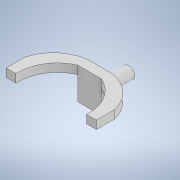
# Autodesk Inventor part: End
Saved by Autodesk Inventor 2022 (Build 260153000, 153)
## iProperties
Created: 2022-01-28
Part Number: End
Material: Generic
Document SubType Name: Modeling
Designer: Alexa
Density: 1 g/cm^3
Appearance: Default
Author: Alexa
Autodesk Inventor part; units mm, degrees
ref_plane "YZ Plane" through (0, 0, 0) normal (1, 0, 0) x (0, 1, 0)
ref_plane "XZ Plane" through (0, 0, 0) normal (0, 1, 0) x (-1, 0, 0)
ref_plane "XY Plane" through (0, 0, 0) normal (0, 0, 1) x (1, 0, 0)
sketch "Sketch1" plane through (0, 0, 0) normal (0, 0, 1) x (1, 0, 0)
  circle A0 centre (0, 0) radius 6
  dimension "d0" = 12
  constraints: 1 centre point, 1 coincident
  measures "d0" diameter of A0
extrude "Extrusion1" add sketch "Sketch1" along normal blind 30
sketch "Sketch2" plane through (0, 0, 30) normal (0, 0, 1) x (1, 0, 0)
  line L0 (0, 0) -> (12, 0)
  line L1 (12, 0) -> (12, 12)
  line L2 (12, 12) -> (0, 12)
  line L3 (0, 12) -> (0, 0)
  line L4 (0, 0) -> (12, 0)
  line L5 (12, 0) -> (12, -12)
  line L6 (12, -12) -> (0, -12)
  line L7 (0, -12) -> (0, 0)
  line L8 (0, 0) -> (-12, 0)
  line L9 (-12, 0) -> (-12, 12)
  line L10 (-12, 12) -> (0, 12)
  line L11 (0, 12) -> (0, 0)
  line L12 (-12, 0) -> (0, 0)
  line L13 (0, 0) -> (0, -12)
  line L14 (0, -12) -> (-12, -12)
  line L15 (-12, -12) -> (-12, 0)
  dimension "d3" = 12
  dimension "d4" = 12
  dimension "d5" = 12
  dimension "d6" = 12
  constraints: 32 end point, 8 parallel, 4 horizontal, 4 perpendicular, 2 point on line
  measures "d3" distance of L2.end L1.end
  measures "d4" distance of L1.end L0.end
  measures "d5" distance of L4.end L5.end
  measures "d6" distance of L9.end L10.end
extrude "Extrusion2" add sketch "Sketch2" along normal blind 10
sketch "Sketch3" plane through (-12, 12, 30) normal (0, 1, 0) x (1, 0, 0)
  line L0 (0, 0) -> (24, 0) projected
  line L1 (0, 0) -> (24, 0)
  line L2 (24, 0) -> (24, -48.9856)
  line L3 (24, -48.9856) -> (0, -48.9856)
  line L4 (0, -48.9856) -> (0, 0)
  line L5 (0, 0) -> (0, -10) projected
  line L6 (0, 0) -> (-24, 0)
  line L7 (-24, 0) -> (-24, -48.9856)
  line L8 (-24, -48.9856) -> (0, -48.9856)
  line L9 (0, -48.9856) -> (0, 0)
  arc A0 (0, -10) -> (-24, -48.9856) centre (15.934, -46.6893) ccw
  line L10 (24, 0) -> (24, -10) projected
  line L11 (24, 0) -> (48, 0)
  line L12 (48, 0) -> (48, -48.9856)
  line L13 (48, -48.9856) -> (24, -48.9856)
  line L14 (24, -48.9856) -> (24, 0)
  line L15 (0, -10) -> (24, -10) projected
  arc A1 (48, -48.9856) -> (24, -10) centre (8.066, -46.6893) ccw
  line L16 (-24, -48.9856) -> (-34, -48.9856)
  line L17 (-34, -48.9856) -> (-34, 0)
  line L18 (-34, 0) -> (-24, 0)
  line L19 (-24, 0) -> (-24, -48.9856)
  line L20 (48, 0) -> (58, 0)
  line L21 (58, 0) -> (58, -48.9856)
  line L22 (58, -48.9856) -> (48, -48.9856)
  line L23 (48, -48.9856) -> (48, 0)
  arc A2 (0, 0) -> (-34, -48.9856) centre (4.9068, -39.6979) ccw
  arc A3 (58, -48.9856) -> (24, 0) centre (19.0932, -39.6979) ccw
  point P0 (12, 30)
  point P1 (58, -30.4102)
  point P2 (-34, -30.4102)
  dimension "d9" = 24
  dimension "d10" = 24
  dimension "d11" = 40
  dimension "d12" = 24
  dimension "d13" = 40
  dimension "d14" = 10
  dimension "d15" = 10
  dimension "d16" = 40
  dimension "d17" = 40
  constraints: 40 end point, 10 parallel, 8 point on circle, 5 horizontal, 5 perpendicular, 4 centre point, 2 point on line
  measures "d9" distance of L2.end L3.end
  measures "d10" distance of L8.end L7.end
  measures "d11" radius of A0
  measures "d12" distance of L12.end L13.end
  measures "d13" radius of A1
  measures "d14" distance of L17.end L18.end
  measures "d15" distance of L21.end L22.end
  measures "d16" radius of A2
  measures "d17" radius of A3
extrude "Extrusion3" add sketch "Sketch3" along normal blind 8.4125 contours L0 L2 L15 L4 | L4 A0 L7 A2 | A3 L12 A1 L2 | L7 A0 L16 L17 A2 | A3 L21 L22 A1 L12
body "Solid1"
